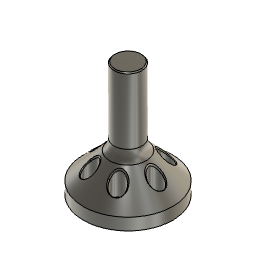
Motor_Shaft v2 (Autodesk Fusion 360 archive; units mm, degrees)
design "Motor_Shaft v2"
part number: Configuration 1
Autodesk Fusion 360 part; units mm, degrees
sketch "Sketch1" plane through (0, 0, 0) normal (0, 0, 1) x (1, 0, 0)
  circle A0 centre (0, 0) radius 22.5
  dimension "d2" = 45
  constraint coincident A0.centre origin
  measures "d2" diameter of A0
extrude "Extrude12" add sketch "Sketch1" along normal blind 6
sketch "Sketch2" plane through (0, 0, 6) normal (0, 0, 1) x (-1, 0, 0)
  circle A0 centre (0, 0) radius 22.5
  circle A1 centre (0, 0) radius 22.5
  circle A2 centre (0, 0) radius 14 construction
  circle A3 centre (14, 0) radius 2
  circle A4 centre (7, 12.1244) radius 2
  circle A5 centre (-7, 12.1244) radius 2
  circle A6 centre (-14, 0) radius 2
  circle A7 centre (-7, -12.1244) radius 2
  circle A8 centre (7, -12.1244) radius 2
  circle A9 centre (14, 0) radius 3.5
  circle A10 centre (7, 12.1244) radius 3.5
  circle A11 centre (-7, 12.1244) radius 3.5
  circle A12 centre (-14, 0) radius 3.5
  circle A13 centre (-7, -12.1244) radius 3.5
  circle A14 centre (7, -12.1244) radius 3.5
  circle A15 centre (0, 0) radius 7
  dimension "d101" = 45
  dimension "d102" = 28
  dimension "d103" = 4
  dimension "d105" = 360
  dimension "d106" = 7
  dimension "d108" = 360
  dimension "d111" = 14
  constraint coincident A0.centre A1.centre
  constraint concentric A1 A2
  constraint coincident A2 A3.centre
  constraint concentric A3 A9
  constraint concentric A1 A15
  measures "d101" diameter of A1
  measures "d102" diameter of A2
  measures "d103" diameter of A3
  measures "d106" diameter of A9
  measures "d111" diameter of A15
extrude "Extrude13" cut sketch "Sketch2" against normal blind 5 contours A3 | A4 | A5 | A6 | A7 | A8
extrude "Extrude14" add sketch "Sketch2" along normal blind 52 contours A15
sketch "Sketch8" plane through (0, 0, 0) normal (1, 0, 0) x (0, 1, 0)
  circle A0 through (-7, 6, 0) (3.5, 6, 6.0622) (3.5, 6, -6.0622)
  circle A1 through (22.5, 6, 0) (-11.25, 6, 19.4856) (-11.25, 6, -19.4856)
  line L0 (-7, 6) -> (-22.5, 6)
  line L1 (-7, 6) -> (-7, 21.5)
  line L2 (-7, 21.5) -> (-22.5, 6)
  dimension "d129" = 15.5
  constraint horizontal L0
  constraint perpendicular L0 L1
  measures "d129" distance of L0.start L1.end
revolve "Revolve2" add sketch "Sketch8" angle 360 about axis through (0, 0, 1.75) along (0, 0, 1)
extrude "Extrude15" cut sketch "Sketch2" along normal blind 15 contours A3 | A4 | A5 | A6 | A7 | A8 | A9 | A10 | A11 | A12 | A13 | A14
sketch "Sketch9" plane through (0, 0, 0) normal (0, 0, 1) x (1, 0, 0)
  circle A0 centre (0, 0) radius 18.25
  dimension "d120" = 36.5
  constraint coincident A0.centre origin
  measures "d120" diameter of A0
extrude "Extrude16" cut sketch "Sketch9" along normal blind 2
chamfer "Chamfer12" distance 0.5 angle 45 1 edges at (6.5263, 2.5313, 58)
chamfer "Chamfer12" distance 0.5 angle 45 1 edges at (-17.015, -6.5995, 2)
chamfer "Chamfer12" distance 0.5 angle 45 12 edges at (-5.1353, -12.8476, 2) (-12.1353, -0.7232, 2) (8.8647, -12.8476, 2) (-5.1353, 11.4011, 2) (8.8647, 11.4011, 2) (15.8647, -0.7232, 2) (-5.1353, -12.8476, 6) (-12.1353, -0.7232, 6) (-5.1353, 11.4011, 6) (8.8647, 11.4011, 6) (15.8647, -0.7232, 6) (8.8647, -12.8476, 6)
chamfer "Chamfer12" distance 0.5 angle 45 6 edges at (14.6341, 3.4421, 13.4666) (10.298, -10.9524, 13.4666) (4.3361, 14.3945, 13.4666) (-4.3361, -14.3945, 13.4666) (-14.6341, -3.4421, 13.4666) (-10.298, 10.9524, 13.4666)
fillet "Fillet5" radius 7.5 1 edges at (6.5263, 2.5313, 21.5)
other "Base Mesh Feature1"
